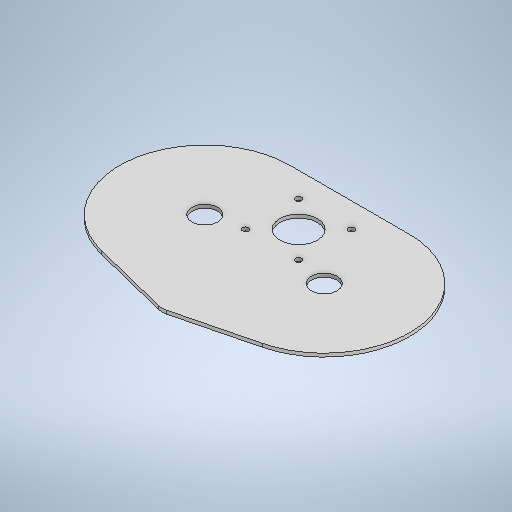
# Autodesk Inventor part: Extruder Frame
Saved by Autodesk Inventor 2025.2 (Build 292293000, 293)
## iProperties
Created: 2025-06-23
Part Number: Extruder Frame
Material: Generic
Document SubType Name: Modeling
Designer: Simon
Density: 1 g/cm^3
Appearance: Default
Author: Simon
Autodesk Inventor part; units mm, degrees
ref_plane "YZ Plane" through (0, 0, 0) normal (1, 0, 0) x (0, 1, 0)
ref_plane "XZ Plane" through (0, 0, 0) normal (0, 1, 0) x (-1, 0, 0)
ref_plane "XY Plane" through (0, 0, 0) normal (0, 0, 1) x (1, 0, 0)
sketch "Sketch1" plane through (0, 0, 0) normal (0, 1, 0) x (-1, 0, 0)
  line L0 (35, 0) -> (-35, 0)
  circle A0 centre (-35, 0) radius 7.5
  circle A1 centre (35, 0) radius 7.5
  circle A2 centre (35, 0) radius 50
  circle A3 centre (-35, 0) radius 50
  line L1 (35, -50) -> (-35, -50)
  line L2 (0, -50) -> (0, -35.5)
  line L3 (15.5, -35.5) -> (-15.5, -35.5)
  line L4 (15.5, -35.5) -> (-15.5, -35.5)
  line L5 (-15.5, -35.5) -> (-15.5, -4.5)
  line L6 (-15.5, -4.5) -> (15.5, -4.5)
  line L7 (15.5, -4.5) -> (15.5, -35.5)
  circle A4 centre (15.5, -35.5) radius 1.8
  circle A5 centre (-15.5, -35.5) radius 1.8
  circle A6 centre (-15.5, -4.5) radius 1.8
  circle A7 centre (15.5, -4.5) radius 1.8
  line L8 (15.5, -35.5) -> (-15.5, -4.5)
  line L9 (-15.5, -4.5) -> (-15.5, -35.5)
  line L10 (-15.5, -35.5) -> (15.5, -4.5)
  circle A8 centre (0, -20) radius 11
  line L11 (0, 0) -> (0, 50)
  circle A9 centre (0, 50) radius 10
  line L12 (47.1461, 48.5023) -> (2.4292, 59.7005)
  line L13 (-2.4292, 59.7005) -> (-47.1461, 48.5023)
  point P0 (0, 35.7071)
  dimension "d0" = 70
  dimension "d1" = 15
  dimension "d2" = 15
  dimension "d3" = 100
  dimension "d4" = 100
  dimension "d5" = 14.5
  dimension "d6" = 31
  dimension "d7" = 31
  dimension "d8" = 3.6
  dimension "d9" = 3.6
  dimension "d10" = 3.6
  dimension "d11" = 3.6
  dimension "d14" = 22
  dimension "d15" = 50
  dimension "d16" = 20
  constraints: 28 end point, 10 centre point, 9 coincident, 6 point on circle, 6 tangent, 4 midpoint, 3 horizontal, 3 vertical, 2 parallel, 2 perpendicular
  measures "d0" distance of L0.start L0.end
  measures "d1" diameter of A0
  measures "d2" diameter of A1
  measures "d3" diameter of A2
  measures "d4" diameter of A3
  measures "d5" distance of L2.start L2.end
  measures "d6" distance of L3.start L3.end
  measures "d7" distance of L4.end L5.end
  measures "d8" diameter of A4
  measures "d9" diameter of A5
  measures "d10" diameter of A6
  measures "d11" diameter of A7
  measures "d14" diameter of A8
  measures "d15" distance of L11.start L11.end
  measures "d16" diameter of A9
extrude "Extrusion1" add sketch "Sketch1" along normal blind 2 contours A3 A7 L6 A6 A2 L0 | L0 L11 A3 | A3 A2 L3 A4 L7 A7 | L0 A2 L11 | L11 A9 L12 A2 | A2 A6 L5 A5 L3 A3 | A3 L13 A9 L11 | A9 | A7 L10 A8 L8 A6 L6 | A3 L2 L1 | L7 A4 L8 A8 A3 A7 | A7 A3 A8 L10 | A6 A2 A8 L10 A5 L5 | L1 L2 A2 | L2 L3 A3 | A2 L3 L2 | L8 A8 A2 A6 | L3 A5 L10 A8 A2 | A2 A8 A3 L3 | A3 A8 L8 A4 L3
body "Solid1"
